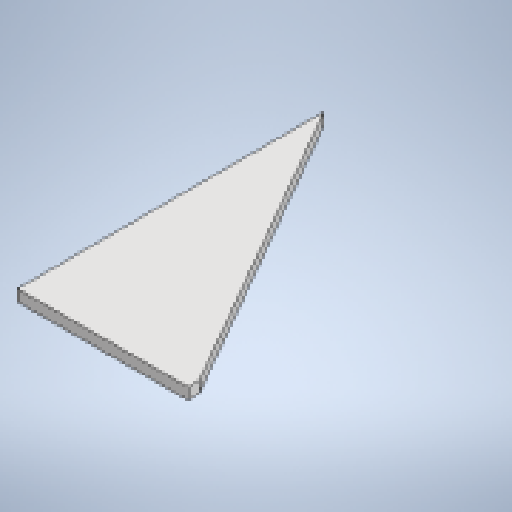
# Autodesk Inventor part: NVPH-324 conductor
Saved by Autodesk Inventor 2025.1 (Build 291241020, 241B)
## iProperties
Created: 2024-12-03
Part Number: NVPH-324 conductor
Material: Generic
Document SubType Name: Sheet Metal
Designer: user
Density: 1 g/cm^3
Flat Pattern Width: 21.6234 cm
Flat Pattern Length: 18.2954 cm
Flat Pattern Area: 395.609 cm^2
Sheet Metal Rule: Default
Sheet Metal Width: 216.234 mm
Sheet Metal Length: 182.954 mm
Sheet Metal Area: 39560.890 mm^2
Appearance: Default
Author: user
Autodesk Inventor part; units mm, degrees
ref_plane "YZ Plane" through (0, 0, 0) normal (1, 0, 0) x (0, 1, 0)
ref_plane "XZ Plane" through (0, 0, 0) normal (0, 1, 0) x (-1, 0, 0)
ref_plane "XY Plane" through (0, 0, 0) normal (0, 0, 1) x (1, 0, 0)
sketch "Sketch3" plane through (0, 0, 0) normal (0, 0, 1) x (1, 0, 0)
  line L0 (0, 0) -> (-150, 0)
  line L1 (-150, 0) -> (-150, 10)
  line L2 (-150, 10) -> (0, 10)
  line L3 (0, 10) -> (0, 0)
  line L4 (0, 10) -> (-150, 269.8076)
  line L5 (-150, 269.8076) -> (-150, 10)
  line L6 (-20, 44.641) -> (-20, 10)
  line L7 (-48, 0) -> (-48, 93.1384)
  line L8 (-150, 216.3134) -> (-119.1151, 216.3134)
  point P0 (-48, 10)
  dimension "d19" = 150
  dimension "d29" = 10
  dimension "d31" = 60
  dimension "d32" = 20
  dimension "d34" = 48
  measures "d19" distance of L0.start L0.end
  measures "d29" distance between parallel lines of L0 L2
  measures "d31" angle of L2 L4
  measures "d32" distance from line of L2.end L6
  measures "d34" distance between parallel lines of L3 L7
extrude "Plate3" add sketch "Sketch3" along normal blind 10 contours L0 L1 L2 L7 | L7 L4 L6 L2 | L2 L5 L8 L4 L7
equation "\"d18\" = Thickness"
equation "\"BendReliefDepth\" = 0.5 * Thickness"
equation "\"Thickness\" = 10"
body "Solid2"
